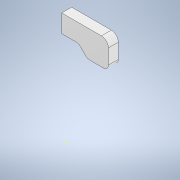
# Autodesk Inventor part: gLOW_rED
Saved by Autodesk Inventor 2022 (Build 260153000, 153)
## iProperties
Created: 2022-02-04
Part Number: gLOW_rED
Material: ABS Plastic
Document SubType Name: Modeling
Designer: joshw
Density: 1.06 g/cm^3
Appearance: Smooth - White
Author: joshw
Autodesk Inventor part; units mm, degrees
ref_plane "YZ Plane" through (0, 0, 0) normal (1, 0, 0) x (0, 1, 0)
ref_plane "XZ Plane" through (0, 0, 0) normal (0, 1, 0) x (-1, 0, 0)
ref_plane "XY Plane" through (0, 0, 0) normal (0, 0, 1) x (1, 0, 0)
sketch "Sketch1" plane through (0, 0, 0) normal (0, 0, 1) x (1, 0, 0)
  line L0 (28.0602, 14.7114) -> (28.0602, 12.4254)
  line L1 (28.0602, 12.4254) -> (29.9461, 12.4254)
  line L2 (30.3951, 12.2394) -> (31.1661, 11.4684)
  line L3 (31.6152, 11.2824) -> (33.3942, 11.2824)
  line L4 (34.0292, 11.9174) -> (34.0292, 13.8224)
  line L5 (33.1402, 14.7114) -> (28.0602, 14.7114)
  arc A0 (34.0292, 13.8224) -> (33.1402, 14.7114) centre (33.1402, 13.8224) ccw
  arc A1 (33.3942, 11.2824) -> (34.0292, 11.9174) centre (33.3942, 11.9174) ccw
  arc A2 (31.1661, 11.4684) -> (31.6152, 11.2824) centre (31.6152, 11.9174) ccw
  arc A3 (30.3951, 12.2394) -> (29.9461, 12.4254) centre (29.9461, 11.7904) ccw
  point P0 (0, 0)
  dimension "d0" = 135
  dimension "d1" = 0.889
  dimension "d2" = 0.635
  dimension "d5" = 5.08
  dimension "d6" = 2.286
  dimension "d7" = 1.886
  dimension "d8" = 1.905
  constraints: 12 end point, 8 point on circle, 8 tangent, 4 centre point, 3 perpendicular, 2 equal radius, 1 horizontal, 1 parallel
  measures "d0" angle of L2 L3
  measures "d1" radius of A0
  measures "d2" radius of A1
  measures "d5" distance of L5.start L0.start
  measures "d6" distance of L0.start L0.end
  measures "d7" distance of L0.end L1.end
  measures "d8" distance of L4.start L4.end
extrude "Extrusion1" add sketch "Sketch1" along normal mid plane 1.27
sketch "Sketch2" plane through (28.0602, 12.4254, -0.635) normal (-1, 0, 0) x (0, 0, 1)
  point P0 (0.635, -12.4254)
sketch "Sketch3" plane through (28.0602, 12.4254, 0.635) normal (-1, 0, 0) x (0, 0, 1)
  line L0 (-1.016, 1.778) -> (-0.762, 1.778)
  line L1 (-0.762, 1.778) -> (-0.762, 0.508)
  line L2 (-0.762, 0.508) -> (-1.016, 0.508)
  line L3 (-1.016, 0.508) -> (-1.016, 1.778)
  line L4 (-1.016, 1.778) -> (-0.762, 0.508) construction
  line L5 (-0.762, 1.778) -> (-1.016, 0.508) construction
  line L6 (-0.635, 2.4021) -> (-0.635, -0.4508)
  line L7 (-1.27, -0.186) -> (0, -0.186) projected
  line L8 (0, 2.286) -> (0, 0) projected
  line L9 (0, 1.143) -> (-1.4315, 1.143)
  line L10 (-0.254, 1.778) -> (-0.508, 1.778)
  line L11 (-0.508, 1.778) -> (-0.508, 0.508)
  line L12 (-0.508, 0.508) -> (-0.254, 0.508)
  line L13 (-0.254, 0.508) -> (-0.254, 1.778)
  line L14 (-0.254, 1.778) -> (-0.508, 0.508) construction
  line L15 (-0.508, 1.778) -> (-0.254, 0.508) construction
  point P0 (-0.635, -12.4254)
  point P1 (-0.889, 1.143)
  point P2 (-0.889, 1.143)
  point P3 (-0.381, 1.143)
  point P4 (-0.381, 1.143)
  dimension "d9" = 0.254
  dimension "d10" = 0.254
  dimension "d11" = 1.27
  constraints: 28 end point, 6 midpoint, 6 symmetric about line, 2 horizontal, 2 parallel, 2 perpendicular, 1 point on line, 1 vertical
  measures "d9" distance of L1.end L2.end
  measures "d10" diameter of L1 L6
  measures "d11" distance between parallel lines of L2 L0
extrude "Extrusion2" cut sketch "Sketch3" against normal blind 4.445
body "Solid1"
